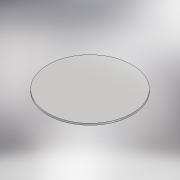
# Autodesk Inventor part: Plateau verre D200
Saved by Autodesk Inventor 2017 (Build 210142000, 142)
## iProperties
Company: FABLAB Frenchmakers
Part Number: Plateau verre D200
Material: Miroir
Document SubType Name: Modeling
Designer: FABLAB Frenchmakers
Density: 2.7 g/cm^3
Appearance: Aluminum - Poli
Mass: 339.292 g
Surface Area: 653.451 cm^2
Volume: 125.664 cm^3
Project: 1420 Vauban 3D XL
Catalog Web Link: http://frenchmakers.com/
Stock Number: 1420-04-03
Hauteur: 4,000 mm
Autodesk Inventor part; units mm, degrees
ref_plane "YZ Plane" through (0, 0, 0) normal (1, 0, 0) x (0, 1, 0)
ref_plane "XZ Plane" through (0, 0, 0) normal (0, 1, 0) x (-1, 0, 0)
ref_plane "XY Plane" through (0, 0, 0) normal (0, 0, 1) x (1, 0, 0)
sketch "Esquisse1" plane through (0, 0, 0) normal (0, 0, 1) x (1, 0, 0)
  circle A0 centre (0, 0) radius 100
  dimension "Diamètre_plateau" = 200
  constraints: 1 centre point, 1 coincident
  measures "Diamètre_plateau" diameter of A0
extrude "Extrusion1" add sketch "Esquisse1" along normal mid plane 4
